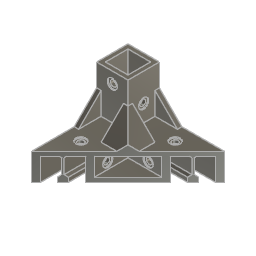
Rear Corner Bracket Top v2 (Autodesk Fusion 360 design; units mm, degrees)
Autodesk Fusion 360 part; units mm, degrees
note: some values were not read from the file. Chosen so that the rebuilt part matches the saved one: which face or edge a step refers to; where a step starts. Set by a fixed rule: which sketch regions a step uses.
sketch "Sketch1" plane through (0, 0, 0) normal (0, 0, 1) x (1, 0, 0)
  line L0 (0, 0) -> (106, 0)
  line L1 (106, 0) -> (106, -106)
  line L2 (106, -106) -> (0, -106)
  line L3 (0, -106) -> (0, 0)
  line L4 (20, 0) -> (20, -106)
  line L5 (0, -20) -> (106, -20)
  line L6 (23.95, 0) -> (23.95, -106)
  line L7 (0, -23.95) -> (4.1623, -23.95)
  line L8 (4.1623, -23.95) -> (106, -23.95)
  line L9 (44.05, 0) -> (44.05, -106)
  line L10 (0, -44.05) -> (106, -44.05)
  line L11 (106, -20) -> (20, -106)
  line L12 (0, -48) -> (106, -48)
  line L13 (48, 0) -> (48, -106)
  line L14 (0, -60) -> (106, -60)
  line L15 (60, 0) -> (60, -106)
  line L16 (0, -56) -> (106, -56)
  line L17 (56, 0) -> (56, -106)
  line L18 (0, -4) -> (106, -4)
  line L19 (4, 0) -> (4, -106)
  line L20 (10, 0) -> (10, -106) construction
  line L21 (0, -10) -> (106, -10) construction
  circle A0 centre (10, -10) radius 2.7
  line L22 (14.2, -12.4249) -> (14.2, -7.5751)
  line L23 (14.2, -7.5751) -> (10, -5.1503)
  line L24 (10, -5.1503) -> (5.8, -7.5751)
  line L25 (5.8, -7.5751) -> (5.8, -12.4249)
  line L26 (5.8, -12.4249) -> (10, -14.8497)
  line L27 (10, -14.8497) -> (14.2, -12.4249)
  line L28 (0, 0) -> (63, -63) construction
  circle A1 centre (10, -48) radius 2.7
  circle A2 centre (48, -10) radius 2.7
  line L29 (52.8497, -10) -> (50.4249, -5.8)
  line L30 (50.4249, -5.8) -> (45.5751, -5.8)
  line L31 (45.5751, -5.8) -> (43.1503, -10)
  line L32 (43.1503, -10) -> (45.5751, -14.2)
  line L33 (45.5751, -14.2) -> (50.4249, -14.2)
  line L34 (50.4249, -14.2) -> (52.8497, -10)
  line L35 (14.2, -50.4249) -> (14.2, -45.5751)
  line L36 (14.2, -45.5751) -> (10, -43.1503)
  line L37 (10, -43.1503) -> (5.8, -45.5751)
  line L38 (5.8, -45.5751) -> (5.8, -50.4249)
  line L39 (5.8, -50.4249) -> (10, -52.8497)
  line L40 (10, -52.8497) -> (14.2, -50.4249)
  line L41 (33.95, -106) -> (33.95, 0) construction
  line L42 (106, -33.95) -> (0, -33.95) construction
  line L43 (106, -76) -> (0, -76) construction
  line L44 (76, -106) -> (76, 0) construction
  circle A3 centre (33.95, -76) radius 2.7
  circle A4 centre (33.95, -76) radius 4.5
  circle A5 centre (76, -33.95) radius 2.7
  circle A6 centre (76, -33.95) radius 4.5
  line L45 (68, 0) -> (68, -106)
  line L46 (0, -68) -> (106, -68)
  line L47 (34.45, -106) -> (34.45, 0)
  line L48 (33.45, -106) -> (33.45, 0)
  line L49 (0, -34.45) -> (106, -34.45)
  line L50 (106, -33.45) -> (0, -33.45)
  line L51 (31.45, 0) -> (31.45, -106)
  line L52 (36.45, -106) -> (36.45, 0)
  line L53 (0, -31.45) -> (106, -31.45)
  line L54 (106, -36.45) -> (0, -36.45)
  point P0 (10, -10)
  point P1 (48, -10)
  point P2 (10, -48)
  dimension "d1" = 106
  dimension "d2" = 106
  dimension "d3" = 20
  dimension "d4" = 20
  dimension "d5" = 3.95
  dimension "d6" = 3.95
  dimension "d7" = 20.1
  dimension "d8" = 20.1
  dimension "d9" = 3.95
  dimension "d10" = 3.95
  dimension "d11" = 60
  dimension "d13" = 60
  dimension "d26" = 4
  dimension "d27" = 4
  dimension "d28" = 4
  dimension "d29" = 4
  dimension "d31" = 10
  dimension "d32" = 10
  dimension "d33" = 5.4
  dimension "d34" = 4.2
  dimension "d35" = 5.4
  dimension "d36" = 5.4
  dimension "d37" = 4.2
  dimension "d38" = 4.2
  dimension "d42" = 10
  dimension "d43" = 10
  dimension "d44" = 30
  dimension "d45" = 30
  dimension "d46" = 5.4
  dimension "d47" = 9
  dimension "d48" = 5.4
  dimension "d49" = 9
  dimension "d115" = 20
  dimension "d116" = 20
  dimension "d118" = 1
  dimension "d120" = 0.5
  dimension "d121" = 1
  dimension "d123" = 0.5
  dimension "d126" = 5
  dimension "d127" = 2.5
  dimension "d128" = 5
  dimension "d129" = 2.5
  constraint horizontal L0
  constraint vertical L1
  constraint horizontal L2
  constraint vertical L3
  constraint coincident L0.start L3.end
  constraint coincident L0 L4.start
  constraint coincident L2 L4.end
  constraint perpendicular L2 L4
  constraint coincident L3 L5.start
  constraint coincident L1 L5.end
  constraint perpendicular L1 L5
  constraint coincident L0 L6.start
  constraint coincident L2 L6.end
  constraint perpendicular L2 L6
  constraint coincident L3 L7.start
  constraint perpendicular L3 L7
  constraint coincident L1 L8.end
  constraint perpendicular L1 L8
  constraint coincident L0 L9.start
  constraint coincident L2 L9.end
  constraint perpendicular L2 L9
  constraint coincident L3 L10.start
  constraint coincident L1 L10.end
  constraint perpendicular L1 L10
  constraint coincident L3 L12.start
  constraint coincident L1 L12.end
  constraint perpendicular L1 L12
  constraint coincident L0 L13.start
  constraint coincident L2 L13.end
  constraint perpendicular L2 L13
  constraint coincident L3 L14.start
  constraint coincident L1 L14.end
  constraint perpendicular L1 L14
  constraint coincident L0 L15.start
  constraint coincident L2 L15.end
  constraint perpendicular L2 L15
  constraint coincident L3 L16.start
  constraint coincident L1 L16.end
  constraint perpendicular L1 L16
  constraint coincident L0 L17.start
  constraint coincident L2 L17.end
  constraint perpendicular L2 L17
  constraint coincident L3 L18.start
  constraint coincident L1 L18.end
  constraint perpendicular L1 L18
  constraint coincident L0 L19.start
  constraint coincident L2 L19.end
  constraint perpendicular L2 L19
  constraint coincident L0 L20.start
  constraint coincident L2 L20.end
  constraint perpendicular L2 L20
  constraint coincident L3 L21.start
  constraint coincident L1 L21.end
  constraint perpendicular L1 L21
  constraint coincident L20 P0
  constraint coincident L21 P0
  constraint coincident P0 A0.centre
  constraint midpoint L11 L28.end
  constraint coincident L12 P2
  constraint coincident L20 P2
  constraint coincident L13 P1
  constraint coincident L21 P1
  constraint coincident P1 A2.centre
  constraint parallel L0 L30
  constraint coincident P2 A1.centre
  constraint parallel L3 L38
  constraint parallel L3 L25
  constraint coincident L2 L41.start
  constraint coincident L0 L41.end
  constraint perpendicular L0 L41
  constraint coincident L1 L42.start
  constraint coincident L3 L42.end
  constraint perpendicular L3 L42
  constraint coincident L1 L43.start
  constraint coincident L3 L43.end
  constraint perpendicular L3 L43
  constraint coincident L2 L44.start
  constraint coincident L0 L44.end
  constraint perpendicular L0 L44
  constraint coincident L43 A3.centre
  constraint coincident L41 A3.centre
  constraint concentric A3 A4
  constraint coincident L44 A5.centre
  constraint coincident L42 A5.centre
  constraint concentric A5 A6
  constraint coincident L0 L45.start
  constraint coincident L2 L45.end
  constraint perpendicular L2 L45
  constraint coincident L3 L46.start
  constraint coincident L1 L46.end
  constraint perpendicular L1 L46
  constraint coincident L2 L47.start
  constraint coincident L0 L47.end
  constraint perpendicular L0 L47
  constraint coincident L2 L48.start
  constraint coincident L0 L48.end
  constraint perpendicular L0 L48
  constraint coincident L3 L49.start
  constraint coincident L1 L49.end
  constraint perpendicular L1 L49
  constraint coincident L1 L50.start
  constraint coincident L3 L50.end
  constraint perpendicular L3 L50
  constraint coincident L0 L51.start
  constraint coincident L2 L51.end
  constraint perpendicular L2 L51
  constraint coincident L2 L52.start
  constraint coincident L0 L52.end
  constraint perpendicular L0 L52
  constraint coincident L3 L53.start
  constraint coincident L1 L53.end
  constraint perpendicular L1 L53
  constraint coincident L1 L54.start
  constraint coincident L3 L54.end
  constraint perpendicular L3 L54
  measures "d1" distance of L0.start L0.end
  measures "d2" distance of L0.start L2.end
  measures "d3" distance of L0 L5
  measures "d4" distance of L3 L4
  measures "d5" distance of L5 L8
  measures "d6" distance of L4 L6
  measures "d7" distance of L6 L9
  measures "d8" distance of L8 L10
  measures "d9" distance of L9 L13
  measures "d10" distance of L10 L12
  measures "d11" distance of L3 L15
  measures "d13" distance of L0 L14
  measures "d26" distance of L15 L17
  measures "d27" distance of L14 L16
  measures "d28" distance of L3 L19
  measures "d29" distance of L0 L18
  measures "d31" distance of L3 L20
  measures "d32" distance of L0 L21
  measures "d33" diameter of A0
  measures "d34" distance of P0 L27
  measures "d35" diameter of A1
  measures "d36" diameter of A2
  measures "d37" distance of P1 L34
  measures "d38" distance of P2 L40
  measures "d42" distance of L8 L42
  measures "d43" distance of L6 L41
  measures "d44" distance of L2 L43
  measures "d45" distance of L1 L44
  measures "d46" diameter of A3
  measures "d47" diameter of A4
  measures "d48" diameter of A5
  measures "d49" diameter of A6
  measures "d115" distance of L13 L45
  measures "d116" distance of L12 L46
  measures "d118" distance of L47 L48
  measures "d120" distance of L41 L47
  measures "d121" distance of L49 L50
  measures "d123" distance of L42 L50
  measures "d126" distance of L51 L52
  measures "d127" distance of L41 L51
  measures "d128" distance of L53 L54
  measures "d129" distance of L42 L54
extrude "Extrude1" add sketch "Sketch1" along normal blind 4 contours L0 L3 L18 L19 | L0 L4 L18 L19 | L3 L5 L18 L19 | L0 L4 L6 L18 | L4 L5 L18 L19 | L3 L5 L7 L19 | L0 L6 L18 L51 | L4 L5 L6 L18 | L4 L5 L7 L8 L19 | L3 L7 L19 L53 | L0 L18 L48 L51 | L5 L6 L18 L51 | L4 L5 L6 L8 | L4 L7 L8 L19 L53 | L3 L19 L50 L53 | L0 L18 L47 L48 | L5 L18 L48 L51 | L5 L6 L8 L51 | L4 L6 L8 L53 | L4 L19 L50 L53 | L3 L19 L49 L50 | L0 L18 L47 L52 | L5 L18 L47 L48 | L5 L8 L48 L51 | L4 L6 L50 L53 | L4 L19 L49 L50 | L3 L19 L49 L54 | L0 L9 L18 L52 | L5 L18 L47 L52 | L5 L8 L47 L48 | L4 L6 L49 L50 | L4 L19 L49 L54 | L3 L10 L19 L54 | L0 L9 L13 L18 | L5 L9 L18 L31 L32 L52 | L5 L8 L47 L52 | L4 L6 L49 L54 | L4 L10 L19 L36 L37 L54 | L3 L10 L12 L19 | L0 L13 L17 L18 | L9 L13 L18 L30 L31 | L5 L8 L9 L52 | L4 L6 L10 L54 | L10 L12 L19 L37 L38 | L3 L12 L16 L19 | L0 L15 L17 L18 | L5 L13 L17 L18 L29 L30 L33 L34 | L9 L13 A2 L30 L31 L32 L33 | L9 L31 L32 | L5 L9 L13 L32 L33 | L5 L8 L9 L13 | L4 L6 L10 L12 | L4 L10 L12 L35 L36 | L10 L36 L37 | L10 L12 A1 L35 L36 L37 L38 | L4 L12 L16 L19 L35 L38 L39 L40 | L3 L14 L16 L19 | L5 L15 L17 L18 | L13 A2 L29 L30 L33 L34 | L5 L8 L13 L17 | L4 L6 L12 L16 | L12 A1 L35 L38 L39 L40 | L4 L14 L16 L19 | L5 L8 L15 L17 | L9 L13 L50 L53 | L10 L12 L48 L51 | L4 L6 L14 L16 | L5 L8 L15 L45 | L13 L17 L50 L53 | L9 L13 L49 L50 | L10 L12 L47 L48 | L12 L16 L48 L51 | L4 L6 L14 L46 | L5 L8 L11 L45 | L15 L17 L50 L53 | L13 L17 L49 L50 | L9 L13 L49 L54 | L10 L12 L47 L52 | L12 L16 L47 L48 | L14 L16 L48 L51 | L4 L6 L11 L46 | L15 L45 L50 L53 | L15 L17 L49 L50 | L13 L17 L49 L54 | L12 L16 L47 L52 | L14 L16 L47 L48 | L14 L46 L48 L51 | A6 L45 L50 L53 | L15 L45 L49 L50 | L15 L17 L49 L54 | L9 L10 L12 L13 | L14 L16 L47 L52 | L14 L46 L47 L48 | A4 L46 L48 L51 | L11 A6 L50 L53 | A6 L45 L49 L50 | A5 A6 L50 L53 | L15 L45 L49 L54 | L10 L12 L13 L17 | L9 L12 L13 L16 | L14 L46 L47 L52 | A4 L46 L47 L48 | A3 A4 L48 L51 | L11 A4 L48 L51 | L11 A6 L49 L50 | A5 A6 L50 L53 | A6 L45 L49 L54 | A5 A6 L49 L50 | A5 L50 L53 | L10 L12 L15 L17 | L12 L13 L16 L17 | L9 L13 L14 L16 | A4 L46 L47 L52 | A3 A4 L47 L48 | A3 A4 L48 L51 | A3 L48 L51 | L11 A4 L47 L48 | L11 A6 L49 L54 | A5 A6 L49 L50 | A5 A6 L49 L54 | A5 L49 L50 | L10 L12 L15 L45 | L12 L15 L16 L17 | L13 L14 L16 L17 | L9 L13 L14 L46 | A3 A4 L47 L52 | A3 L47 L48 | A3 A4 L47 L48 | L11 A4 L47 L52 | A5 A6 L49 L54 | L10 L11 L12 L45 | A5 L49 L54 | L12 L15 L16 L45 | L14 L15 L16 L17 | L13 L14 L17 L46 | L9 L11 L13 L46 | A3 L47 L52 | A3 A4 L47 L52 | L11 L12 L16 L45 | L11 L14 L15 L16 L45 | L11 L14 L15 L17 L46 | L11 L13 L17 L46 | L11 L16 L45 | L11 L14 L15 | L11 L17 L46 | L22 L23 L24 L25 L26 L27 makes body 1 at (27.3167, -14.3817, 0) makes body 2 at (56.6833, -56.6833, 0) makes body 3 at (33.1167, -76.05, 0) makes body 4 at (76.05, -33.1167, 0)
extrude "Extrude5" add sketch "Sketch1" along normal blind 4 from surface at 4 contours L0 L3 L18 L19 | L0 L4 L18 L19 | L3 L5 L18 L19 | L0 L4 L6 L18 | L4 L5 L18 L19 | L3 L5 L7 L19 | L0 L6 L18 L51 | L4 L5 L6 L18 | L4 L5 L7 L8 L19 | L3 L7 L19 L53 | L0 L18 L48 L51 | L5 L6 L18 L51 | L4 L5 L6 L8 | L4 L7 L8 L19 L53 | L3 L19 L50 L53 | L0 L18 L47 L48 | L5 L18 L48 L51 | L5 L6 L8 L51 | L4 L6 L8 L53 | L4 L19 L50 L53 | L3 L19 L49 L50 | L0 L18 L47 L52 | L5 L18 L47 L48 | L5 L8 L48 L51 | L4 L6 L50 L53 | L4 L19 L49 L50 | L3 L19 L49 L54 | L0 L9 L18 L52 | L5 L18 L47 L52 | L5 L8 L47 L48 | L4 L6 L49 L50 | L4 L19 L49 L54 | L3 L10 L19 L54 | L0 L9 L13 L18 | L5 L9 L18 L31 L32 L52 | L5 L8 L47 L52 | L4 L6 L49 L54 | L4 L10 L19 L36 L37 L54 | L3 L10 L12 L19 | L0 L13 L17 L18 | L9 L13 L18 L30 L31 | L5 L8 L9 L52 | L4 L6 L10 L54 | L10 L12 L19 L37 L38 | L3 L12 L16 L19 | L0 L15 L17 L18 | L5 L13 L17 L18 L29 L30 L33 L34 | L5 L9 L13 L32 L33 | L5 L8 L9 L13 | L4 L6 L10 L12 | L4 L10 L12 L35 L36 | L4 L12 L16 L19 L35 L38 L39 L40 | L3 L14 L16 L19 | L5 L15 L17 L18 | L5 L8 L13 L17 | L4 L6 L12 L16 | L4 L14 L16 L19 | L5 L8 L15 L17 | L4 L6 L14 L16 | L5 L8 L15 L45 | L9 L13 L49 L50 | L10 L12 L47 L48 | L4 L6 L14 L46 | L5 L8 L11 L45 | L13 L17 L49 L50 | L12 L16 L47 L48 | L4 L6 L11 L46 | L15 L17 L49 L50 | L14 L16 L47 L48 | L15 L45 L49 L50 | L9 L10 L12 L13 | L14 L46 L47 L48 | A6 L45 L49 L50 | L10 L12 L13 L17 | L9 L12 L13 L16 | A4 L46 L47 L48 | L11 A6 L49 L50 | A5 A6 L49 L50 | L10 L12 L15 L17 | L9 L13 L14 L16 | A3 A4 L47 L48 | L11 A4 L47 L48 | A5 A6 L49 L50 | A5 L49 L50 | L10 L12 L15 L45 | L9 L13 L14 L46 | A3 L47 L48 | A3 A4 L47 L48 | L10 L11 L12 L45 | L9 L11 L13 L46 bodies 3 1 4 2
extrude "Extrude2" add sketch "Sketch1" along normal blind 12 from surface at 8 contours L0 L3 L18 L19 | L0 L4 L18 L19 | L3 L5 L18 L19 | L0 L4 L6 L18 | L4 L5 L18 L19 | L3 L5 L7 L19 | L0 L6 L18 L51 | L4 L5 L6 L18 | L4 L5 L7 L8 L19 | L3 L7 L19 L53 | L0 L18 L48 L51 | L4 L5 L6 L8 | L3 L19 L50 L53 | L0 L18 L47 L48 | L5 L6 L8 L51 | L4 L6 L8 L53 | L3 L19 L49 L50 | L0 L18 L47 L52 | L5 L8 L48 L51 | L4 L6 L50 L53 | L3 L19 L49 L54 | L0 L9 L18 L52 | L5 L8 L47 L48 | L4 L6 L49 L50 | L3 L10 L19 L54 | L0 L9 L13 L18 | L5 L8 L47 L52 | L4 L6 L49 L54 | L3 L10 L12 L19 | L0 L13 L17 L18 | L5 L8 L9 L52 | L4 L6 L10 L54 | L3 L12 L16 L19 | L0 L15 L17 L18 | L5 L8 L9 L13 | L4 L6 L10 L12 | L3 L14 L16 L19 | L5 L15 L17 L18 | L5 L8 L13 L17 | L4 L6 L12 L16 | L4 L14 L16 L19 | L5 L8 L15 L17 | L4 L6 L14 L16 | L5 L8 L15 L45 | L9 L13 L49 L50 | L10 L12 L47 L48 | L4 L6 L14 L46 | L5 L8 L11 L45 | L13 L17 L49 L50 | L12 L16 L47 L48 | L4 L6 L11 L46 | L15 L17 L49 L50 | L14 L16 L47 L48 | L15 L45 L49 L50 | L9 L10 L12 L13 | L14 L46 L47 L48 | A6 L45 L49 L50 | L10 L12 L13 L17 | L9 L12 L13 L16 | A4 L46 L47 L48 | L11 A6 L49 L50 | A5 A6 L49 L50 | L10 L12 L15 L17 | L9 L13 L14 L16 | A3 A4 L47 L48 | L11 A4 L47 L48 | A5 A6 L49 L50 | A5 L49 L50 | L10 L12 L15 L45 | L9 L13 L14 L46 | A3 L47 L48 | A3 A4 L47 L48 | L10 L11 L12 L45 | L9 L11 L13 L46 bodies 3 1 4 2
extrude "Extrude3" add sketch "Sketch1" along normal blind 4 from surface at 20 contours L0 L3 L18 L19 | L0 L4 L18 L19 | L3 L5 L18 L19 | L0 L4 L6 L18 | L4 L5 L18 L19 | L3 L5 L7 L19 | L0 L6 L18 L51 | L4 L5 L6 L18 | L4 L5 L7 L8 L19 | L3 L7 L19 L53 | L0 L18 L48 L51 | L4 L5 L6 L8 | L3 L19 L50 L53 | L0 L18 L47 L48 | L5 L6 L8 L51 | L4 L6 L8 L53 | L3 L19 L49 L50 | L0 L18 L47 L52 | L5 L8 L48 L51 | L4 L6 L50 L53 | L3 L19 L49 L54 | L0 L9 L18 L52 | L5 L8 L47 L48 | L4 L6 L49 L50 | L3 L10 L19 L54 | L0 L9 L13 L18 | L5 L8 L47 L52 | L4 L6 L49 L54 | L3 L10 L12 L19 | L0 L13 L17 L18 | L5 L8 L9 L52 | L4 L6 L10 L54 | L3 L12 L16 L19 | L0 L15 L17 L18 | L5 L8 L9 L13 | L4 L6 L10 L12 | L3 L14 L16 L19 | L5 L15 L17 L18 | L5 L8 L13 L17 | L8 L9 L13 L53 | L6 L10 L12 L51 | L4 L6 L12 L16 | L4 L14 L16 L19 | L5 L8 L15 L17 | L8 L13 L17 L53 | L9 L13 L50 L53 | L10 L12 L48 L51 | L6 L12 L16 L51 | L4 L6 L14 L16 | L5 L8 L15 L45 | L8 L15 L17 L53 | L13 L17 L50 L53 | L9 L13 L49 L50 | L10 L12 L47 L48 | L12 L16 L48 L51 | L6 L14 L16 L51 | L4 L6 L14 L46 | L5 L8 L11 L45 | L8 L15 L45 L53 | L15 L17 L50 L53 | L13 L17 L49 L50 | L9 L13 L49 L54 | L10 L12 L47 L52 | L12 L16 L47 L48 | L14 L16 L48 L51 | L6 L14 L46 L51 | L4 L6 L11 L46 | L8 L11 A6 L45 L53 | L15 L45 L50 L53 | L15 L17 L49 L50 | L13 L17 L49 L54 | L9 L10 L13 L54 | L9 L10 L12 L52 | L12 L16 L47 L52 | L14 L16 L47 L48 | L14 L46 L48 L51 | L6 L11 A4 L46 L51 | A6 L45 L50 L53 | L15 L45 L49 L50 | L15 L17 L49 L54 | L10 L13 L17 L54 | L9 L10 L12 L13 | L9 L12 L16 L52 | L14 L16 L47 L52 | L14 L46 L47 L48 | A4 L46 L48 L51 | L11 A6 L50 L53 | A6 L45 L49 L50 | A5 A6 L50 L53 | A5 A6 L53 | L15 L45 L49 L54 | L10 L15 L17 L54 | L10 L12 L13 L17 | L9 L12 L13 L16 | L9 L14 L16 L52 | L14 L46 L47 L52 | A4 L46 L47 L48 | A3 A4 L51 | A3 A4 L48 L51 | L11 A4 L48 L51 | L11 A6 L49 L50 | A5 A6 L50 L53 | A6 L45 L49 L54 | A5 A6 L49 L50 | A5 L50 L53 | A5 L53 | L10 L15 L45 L54 | L10 L12 L15 L17 | L12 L13 L16 L17 | L9 L13 L14 L16 | L9 L14 L46 L52 | A4 L46 L47 L52 | A3 A4 L47 L48 | A3 A4 L48 L51 | A3 L51 | A3 L48 L51 | L11 A4 L47 L48 | L11 A6 L49 L54 | A5 A6 L49 L50 | L10 L11 A6 L45 L54 | A5 A6 L49 L54 | A5 L49 L50 | L10 L12 L15 L45 | L12 L15 L16 L17 | L13 L14 L16 L17 | L9 L13 L14 L46 | L9 L11 A4 L46 L52 | A3 A4 L47 L52 | A3 L47 L48 | A3 A4 L47 L48 | L11 A4 L47 L52 | A5 A6 L49 L54 | L10 L11 L12 L45 | A5 A6 L54 | A5 L49 L54 | L12 L15 L16 L45 | L14 L15 L16 L17 | L13 L14 L17 L46 | L9 L11 L13 L46 | A3 A4 L52 | A3 L47 L52 | A3 A4 L47 L52 | L11 L12 L16 L45 | A5 L54 | L11 L14 L15 L16 L45 | L11 L14 L15 L17 L46 | L11 L13 L17 L46 | A3 L52 | L11 L16 L45 | L11 L14 L15 | L11 L17 L46 | A0 | L22 L23 L24 L25 L26 L27 bodies 1 2
extrude "Extrude16" add sketch "Sketch1" along normal blind 20 from surface at 24 contours L4 L5 L6 L8 | L5 L6 L8 L51 | L4 L6 L8 L53 | L5 L8 L48 L51 | L4 L6 L50 L53 | L5 L8 L47 L48 | L4 L6 L49 L50 | L5 L8 L47 L52 | L4 L6 L49 L54 | L5 L8 L9 L52 | L4 L6 L10 L54 | L5 L8 L9 L13 | L4 L6 L10 L12 | L5 L8 L13 L17 | L8 L9 L13 L53 | L6 L10 L12 L51 | L4 L6 L12 L16 | L5 L8 L15 L17 | L9 L13 L50 L53 | L10 L12 L48 L51 | L4 L6 L14 L16 | L5 L8 L15 L45 | L9 L13 L49 L50 | L10 L12 L47 L48 | L4 L6 L14 L46 | L9 L13 L49 L54 | L10 L12 L47 L52 | L9 L10 L13 L54 | L9 L10 L12 L52 | L9 L10 L12 L13 | L10 L12 L13 L17 | L9 L12 L13 L16 | L10 L12 L15 L17 | L12 L13 L16 L17 | L9 L13 L14 L16 | L10 L12 L15 L45 | L12 L15 L16 L17 | L13 L14 L16 L17 | L9 L13 L14 L46 | L12 L15 L16 L45 | L14 L15 L16 L17 | L13 L14 L17 L46 | L11 L14 L15 L16 L45 | L11 L14 L15 L17 L46 | L11 L14 L15 bodies 1
combine "Combine1" operation add target body 1 tool bodies 3 4
extrude "Extrude4" add sketch "Sketch1" along normal blind 20 from surface at 44 contours L4 L5 L6 L8 | L5 L6 L8 L51 | L4 L6 L8 L53 | L5 L8 L48 L51 | L4 L6 L50 L53 | L5 L8 L47 L48 | L4 L6 L49 L50 | L5 L8 L47 L52 | L4 L6 L49 L54 | L5 L8 L9 L52 | L4 L6 L10 L54 | L5 L8 L9 L13 | L4 L6 L10 L12 | L8 L9 L13 L53 | L6 L10 L12 L51 | L9 L13 L50 L53 | L10 L12 L48 L51 | L9 L13 L49 L50 | L10 L12 L47 L48 | L9 L13 L49 L54 | L10 L12 L47 L52 | L9 L10 L13 L54 | L9 L10 L12 L52 | L9 L10 L12 L13 bodies 1
extrude "Extrude6" cut sketch "Sketch1" along normal up to surface (3.8 mm away) from surface at 20.2 contours A5 L50 L53 | A5 L53 | A3 L51 | A3 L48 L51 | A5 L49 L50 | A3 L47 L48 | A5 L49 L54 | A3 L47 L52 | A5 L54 | A3 L52 bodies 1
extrude "Extrude17" cut sketch "Sketch1" against normal blind 1 from surface at 20 contours A5 L50 L53 | A5 L53 | A3 L51 | A3 L48 L51 | A5 L49 L50 | A3 L47 L48 | A5 L49 L54 | A3 L47 L52 | A5 L54 | A3 L52 bodies 1
extrude "Extrude7" cut sketch "Sketch1" against normal blind 1 from surface at 24 contours A5 A6 L50 L53 | A5 A6 L53 | A3 A4 L51 | A3 A4 L48 L51 | A5 A6 L50 L53 | A5 A6 L49 L50 | A5 L50 L53 | A5 L53 | A3 A4 L47 L48 | A3 A4 L48 L51 | A3 L51 | A3 L48 L51 | A5 A6 L49 L50 | A5 A6 L49 L54 | A5 L49 L50 | A3 A4 L47 L52 | A3 L47 L48 | A3 A4 L47 L48 | A5 A6 L49 L54 | A5 A6 L54 | A5 L49 L54 | A3 A4 L52 | A3 L47 L52 | A3 A4 L47 L52 | A5 L54 | A3 L52 bodies 1
sketch "Sketch2" plane through (0, 0, 0) normal (1, 0, 0) x (0, 1, 0)
  line L0 (0, 0) -> (-106, 0)
  line L1 (-106, 0) -> (-106, 64)
  line L2 (-106, 64) -> (0, 64)
  line L3 (0, 64) -> (0, 0)
  line L4 (-20, 64) -> (-20, 0) construction
  line L5 (-106, 20) -> (0, 20) construction
  line L6 (0, 10) -> (-106, 10) construction
  line L7 (-48, 64) -> (-48, 0) construction
  line L8 (-34, 64) -> (-34, 0) construction
  line L9 (-20, 39) -> (-48, 39) construction
  line L10 (-82, 64) -> (-82, 0) construction
  line L11 (-44, 64) -> (-44, 0) construction
  line L12 (-66, 64) -> (-66, 0) construction
  circle A0 centre (-34, 39) radius 2.7
  circle A1 centre (-34, 39) radius 4.5
  circle A2 centre (-66, 10) radius 2.7
  circle A3 centre (-66, 10) radius 4.5
  dimension "d56" = 106
  dimension "d57" = 64
  dimension "d58" = 20
  dimension "d59" = 20
  dimension "d61" = 10
  dimension "d62" = 28
  dimension "d63" = 14
  dimension "d64" = 25
  dimension "d65" = 24
  dimension "d66" = 38
  dimension "d67" = 16
  dimension "d68" = 5.4
  dimension "d69" = 9
  dimension "d70" = 5.4
  dimension "d71" = 9
  constraint horizontal L0
  constraint vertical L1
  constraint horizontal L2
  constraint vertical L3
  constraint coincident L0.start L3.end
  constraint coincident L2 L4.start
  constraint coincident L0 L4.end
  constraint perpendicular L0 L4
  constraint coincident L1 L5.start
  constraint coincident L3 L5.end
  constraint perpendicular L3 L5
  constraint coincident L3 L6.start
  constraint coincident L1 L6.end
  constraint perpendicular L1 L6
  constraint coincident L2 L7.start
  constraint coincident L0 L7.end
  constraint perpendicular L0 L7
  constraint coincident L2 L8.start
  constraint coincident L0 L8.end
  constraint perpendicular L0 L8
  constraint coincident L4 L9.start
  constraint coincident L7 L9.end
  constraint perpendicular L7 L9
  constraint coincident L2 L10.start
  constraint coincident L0 L10.end
  constraint perpendicular L0 L10
  constraint coincident L2 L11.start
  constraint coincident L0 L11.end
  constraint perpendicular L0 L11
  constraint coincident L2 L12.start
  constraint coincident L0 L12.end
  constraint perpendicular L0 L12
  constraint midpoint L9 A0.centre
  constraint concentric A0 A1
  constraint coincident L6 A2.centre
  constraint coincident L12 A2.centre
  constraint concentric A2 A3
  measures "d56" distance of L0.start L0.end
  measures "d57" distance of L0.start L2.end
  measures "d58" distance of L3 L4
  measures "d59" distance of L0 L5
  measures "d61" distance of L0 L6
  measures "d62" distance of L4 L7
  measures "d63" distance of L4 L8
  measures "d64" distance of L2 L9
  measures "d65" distance of L1 L10
  measures "d66" distance of L10 L11
  measures "d67" distance of L10 L12
  measures "d68" diameter of A0
  measures "d69" diameter of A1
  measures "d70" diameter of A2
  measures "d71" diameter of A3
extrude "Extrude8" cut sketch "Sketch2" along normal up to surface (3.95 mm away) from surface at 44.05 contours A2 bodies 1
extrude "Extrude9" cut sketch "Sketch2" against normal blind 1 from surface at 48 contours A3 bodies 1
extrude "Extrude10" cut sketch "Sketch2" against normal up to surface (3.95 mm away) from surface at 48 contours A0 bodies 1
extrude "Extrude11" cut sketch "Sketch2" against normal blind 1 from surface at 48 contours A1 bodies 1
sketch "Sketch3" plane through (0, 0, 0) normal (0, 1, 0) x (1, 0, 0)
  line L0 (106, -54) -> (0, -54) construction
  line L1 (48, 0) -> (48, -64) construction
  line L2 (82, -10) -> (44, -10) construction
  line L3 (0, 0) -> (106, 0)
  circle A0 centre (34, -54) radius 2.7
  line L4 (44, 0) -> (44, -64) construction
  line L5 (34, 0) -> (34, -64) construction
  line L6 (20, 0) -> (20, -64) construction
  circle A1 centre (34, -54) radius 4.5
  line L7 (66, 0) -> (66, -64) construction
  line L8 (106, 0) -> (106, -64)
  circle A2 centre (66, -10) radius 4.5
  circle A3 centre (66, -10) radius 2.7
  line L9 (82, 0) -> (82, -64) construction
  line L10 (0, -44) -> (106, -44) construction
  line L11 (0, -64) -> (0, 0)
  line L12 (106, -64) -> (0, -64)
  point P0 (106, -64)
  dimension "d84" = 106
  dimension "d85" = 64
  dimension "d86" = 24
  dimension "d87" = 20
  dimension "d88" = 10
  dimension "d89" = 38
  dimension "d90" = 16
  dimension "d91" = 10
  dimension "d92" = 20
  dimension "d93" = 28
  dimension "d94" = 14
  dimension "d95" = 5.4
  dimension "d96" = 9
  dimension "d97" = 5.4
  dimension "d98" = 9
  constraint horizontal L12
  constraint vertical L11
  constraint horizontal L3
  constraint vertical L8
  constraint coincident P0 L8.end
  constraint coincident L9.start L3
  constraint coincident L9.end L12
  constraint perpendicular L9 L12
  constraint coincident L10.start L11
  constraint coincident L10.end L8
  constraint perpendicular L8 L10
  constraint coincident L0.start L8
  constraint coincident L0.end L11
  constraint perpendicular L0 L11
  constraint coincident L4.start L3
  constraint coincident L4.end L12
  constraint perpendicular L4 L12
  constraint coincident L7.start L3
  constraint coincident L7.end L12
  constraint perpendicular L7 L12
  constraint coincident L2.start L9
  constraint coincident L2.end L4
  constraint perpendicular L2 L4
  constraint coincident L6.start L3
  constraint coincident L6.end L12
  constraint perpendicular L6 L12
  constraint coincident L1.start L3
  constraint coincident L1.end L12
  constraint perpendicular L1 L12
  constraint coincident L5.start L3
  constraint coincident L5.end L12
  constraint perpendicular L5 L12
  constraint concentric A2 A3
  constraint coincident A0.centre L0
  constraint coincident A0.centre L5
  constraint concentric A0 A1
  constraint coincident L3.start L11.end
  constraint coincident A2.centre L7
  measures "d84" distance of P0 L11.start
  measures "d85" distance of P0 L3.end
  measures "d86" distance of L8 L9
  measures "d87" distance of L10 L12
  measures "d88" distance of L0 L12
  measures "d89" distance of L4 L9
  measures "d90" distance of L7 L9
  measures "d91" distance of L2 L3
  measures "d92" distance of L6 L11
  measures "d93" distance of L1 L6
  measures "d94" distance of L5 L6
  measures "d95" diameter of A3
  measures "d96" diameter of A2
  measures "d97" diameter of A0
  measures "d98" diameter of A1
extrude "Extrude12" cut sketch "Sketch3" against normal up to surface (3.95 mm away) from surface at -44.05 contours A3 bodies 1
extrude "Extrude13" cut sketch "Sketch3" along normal blind 1 from surface at -48 contours A2 bodies 1
extrude "Extrude14" cut sketch "Sketch3" along normal up to surface (3.95 mm away) from surface at -48 contours A0 bodies 1
extrude "Extrude15" cut sketch "Sketch3" along normal blind 1 from surface at -48 contours A1 bodies 1
chamfer "Chamfer2" distance 19.9999 angle 45 2 edges at (0, -30, 24) (30, 0, 24) on bodies 1
fillet "Fillet1" radius 5 3 edges at (0, 0, 2) (0, -60, 2) (60, 0, 2) on bodies 1
chamfer "Chamfer3" distance 20 angle 45 4 edges at (68, -21.975, 44) (68, -51.025, 44) (51.025, -68, 44) (21.975, -68, 44) on bodies 1
chamfer "Chamfer5" distance 1 angle 45 8 edges at (85.1016, -34.45, 20) (85.6016, -33.45, 20) (58.6984, -33.45, 20) (58.6984, -34.45, 20) (33.45, -85.6016, 20) (34.45, -85.1016, 20) (34.45, -58.6984, 20) (33.45, -58.6984, 20) on bodies 1
chamfer "Chamfer6" distance 2 angle 45 4 edges at (68.3, -33.45, 4) (67.8, -34.45, 4) (34.45, -67.8, 4) (33.45, -68.3, 4) on bodies 1
